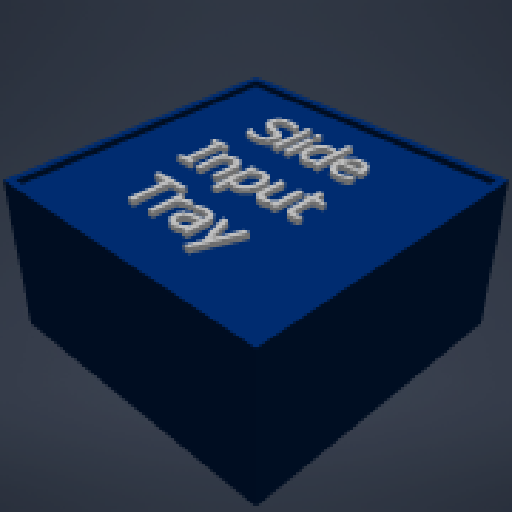
# Autodesk Inventor part: Slide Export Tray
Saved by Autodesk Inventor 2025.1 (Build 291241000, 241)
## iProperties
Created: 2024-10-31
Part Number: Slide Export Tray
Material: Generic
Document SubType Name: Modeling
Designer: jerem
Density: 1 g/cm^3
Appearance: Default
Author: jerem
Autodesk Inventor part; units mm, degrees
ref_plane "YZ Plane" through (0, 0, 0) normal (1, 0, 0) x (0, 1, 0)
ref_plane "XZ Plane" through (0, 0, 0) normal (0, 1, 0) x (-1, 0, 0)
ref_plane "XY Plane" through (0, 0, 0) normal (0, 0, 1) x (1, 0, 0)
sketch "Sketch1" plane through (0, 0, 0) normal (0, 1, 0) x (-1, 0, 0)
  line L0 (-50, 50) -> (50, 50)
  line L1 (50, 50) -> (50, -50)
  line L2 (50, -50) -> (-50, -50)
  line L3 (-50, -50) -> (-50, 50)
  line L4 (-50, 50) -> (50, -50) construction
  line L5 (50, 50) -> (-50, -50) construction
  line L6 (-47.5, 47.5) -> (47.5, 47.5)
  line L7 (47.5, 47.5) -> (47.5, -47.5)
  line L8 (47.5, -47.5) -> (-47.5, -47.5)
  line L9 (-47.5, -47.5) -> (-47.5, 47.5)
  line L10 (-47.5, 47.5) -> (47.5, -47.5) construction
  line L11 (47.5, 47.5) -> (-47.5, -47.5) construction
  point P0 (0, 0)
  dimension "d0" = 100
  dimension "d1" = 100
  dimension "d3" = 95
  constraints: 24 end point, 4 midpoint, 4 parallel, 2 horizontal, 2 perpendicular, 1 point on line
  measures "d0" distance of L1.end L2.end
  measures "d1" distance of L0.end L1.end
  measures "d3" distance of L7.end L8.end
extrude "Extrusion1" add sketch "Sketch1" along normal blind 50 contours L0 L1 L2 L3 | L6 L7 L8 L9
extrude "Extrusion2" add sketch "Sketch1" along normal blind 2 from surface at 50
sketch "Sketch2" plane through (0, 50, 0) normal (0, 1, 0) x (1, 0, 0)
  line L0 (-37.0883, 25.1556) -> (31.9282, 25.1556) construction
  line L1 (31.9282, 25.1556) -> (31.9282, -26.4456) construction
  line L2 (31.9282, -26.4456) -> (-37.0883, -26.4456) construction
  line L3 (-37.0883, -26.4456) -> (-37.0883, 25.1556) construction
  spline S0 degree 2 poles (-18.4674, 18.0229) (-20.0963, 18.0229) (-22.3815, 18.7036) (-23.3904, 19.1899) knots 0 0 0 1 2 2 2
  line L4 (-23.3904, 19.1899) -> (-23.3904, 21.6939)
  line L5 (-23.3904, 21.6939) -> (-23.2446, 21.6939)
  spline S1 degree 2 poles (-23.2446, 21.6939) (-22.26, 20.7701) (-19.7681, 19.749) (-18.6133, 19.749) knots 0 0 0 1 2 2 2
  spline S2 degree 2 poles (-18.6133, 19.749) (-16.9601, 19.749) (-15.2705, 21.1226) (-15.2705, 22.2531) knots 0 0 0 1 2 2 2
  spline S3 degree 2 poles (-15.2705, 22.2531) (-15.2705, 23.1526) (-16.1579, 24.2709) (-17.1181, 24.5505) knots 0 0 0 1 2 2 2
  spline S4 degree 2 poles (-17.1181, 24.5505) (-17.811, 24.745) (-18.9658, 25.0124) (-19.8288, 25.2312) knots 0 0 0 1 2 2 2
  spline S5 degree 2 poles (-19.8288, 25.2312) (-20.6068, 25.4378) (-21.8345, 26.0578) (-22.3086, 26.5561) knots 0 0 0 1 2 2 2
  spline S6 degree 2 poles (-22.3086, 26.5561) (-22.7705, 27.0545) (-23.281, 28.3916) (-23.281, 29.2668) knots 0 0 0 1 2 2 2
  spline S7 degree 2 poles (-23.281, 29.2668) (-23.281, 31.0902) (-20.4366, 33.5578) (-18.2365, 33.5578) knots 0 0 0 1 2 2 2
  spline S8 degree 2 poles (-18.2365, 33.5578) (-16.9723, 33.5578) (-14.7356, 33.0594) (-13.7754, 32.5853) knots 0 0 0 1 2 2 2
  line L6 (-13.7754, 32.5853) -> (-13.7754, 30.2028)
  line L7 (-13.7754, 30.2028) -> (-13.9212, 30.2028)
  spline S9 degree 2 poles (-13.9212, 30.2028) (-14.6384, 30.8592) (-16.875, 31.8317) (-18.1027, 31.8317) knots 0 0 0 1 2 2 2
  spline S10 degree 2 poles (-18.1027, 31.8317) (-19.4885, 31.8317) (-21.2024, 30.531) (-21.2024, 29.4735) knots 0 0 0 1 2 2 2
  spline S11 degree 2 poles (-21.2024, 29.4735) (-21.2024, 28.5253) (-20.1935, 27.3949) (-19.2454, 27.1396) knots 0 0 0 1 2 2 2
  spline S12 degree 2 poles (-19.2454, 27.1396) (-18.6133, 26.9694) (-16.7778, 26.5318) (-16.17, 26.3495) knots 0 0 0 1 2 2 2
  spline S13 degree 2 poles (-16.17, 26.3495) (-14.6262, 25.8754) (-13.1919, 23.967) (-13.1919, 22.5691) knots 0 0 0 1 2 2 2
  spline S14 degree 2 poles (-13.1919, 22.5691) (-13.1919, 21.6818) (-13.9091, 19.98) (-14.5533, 19.3843) knots 0 0 0 1 2 2 2
  spline S15 degree 2 poles (-14.5533, 19.3843) (-15.2705, 18.7279) (-17.0938, 18.0229) (-18.4674, 18.0229) knots 0 0 0 1 2 2 2
  line L8 (-9.375, 18.2903) -> (-11.2713, 18.2903)
  line L9 (-11.2713, 18.2903) -> (-11.2713, 33.9589)
  line L10 (-11.2713, 33.9589) -> (-9.375, 33.9589)
  line L11 (-9.375, 33.9589) -> (-9.375, 18.2903)
  line L12 (-4.6587, 18.2903) -> (-6.5549, 18.2903)
  line L13 (-6.5549, 18.2903) -> (-6.5549, 29.5464)
  line L14 (-6.5549, 29.5464) -> (-4.6587, 29.5464)
  line L15 (-4.6587, 29.5464) -> (-4.6587, 18.2903)
  line L16 (-4.525, 31.4184) -> (-6.6765, 31.4184)
  line L17 (-6.6765, 31.4184) -> (-6.6765, 33.3876)
  line L18 (-6.6765, 33.3876) -> (-4.525, 33.3876)
  line L19 (-4.525, 33.3876) -> (-4.525, 31.4184)
  line L20 (6.7797, 18.2903) -> (4.8835, 18.2903)
  line L21 (4.8835, 18.2903) -> (4.8835, 19.433)
  spline S16 degree 2 poles (4.8835, 19.433) (4.4459, 19.0683) (3.8016, 18.5821) (3.364, 18.3754) knots 0 0 0 1 2 2 2
  spline S17 degree 2 poles (3.364, 18.3754) (2.9629, 18.1809) (2.0998, 17.9743) (1.5285, 17.9743) knots 0 0 0 1 2 2 2
  spline S18 degree 2 poles (1.5285, 17.9743) (0.6047, 17.9743) (-0.9512, 18.7401) (-1.4982, 19.4816) knots 0 0 0 1 2 2 2
  spline S19 degree 2 poles (-1.4982, 19.4816) (-2.0452, 20.2231) (-2.653, 22.4111) (-2.653, 23.8333) knots 0 0 0 1 2 2 2
  spline S20 degree 2 poles (-2.653, 23.8333) (-2.653, 25.3163) (-1.8872, 27.48) (-1.2186, 28.2944) knots 0 0 0 1 2 2 2
  spline S21 degree 2 poles (-1.2186, 28.2944) (-0.5987, 29.0237) (1.1396, 29.8625) (2.0998, 29.8625) knots 0 0 0 1 2 2 2
  spline S22 degree 2 poles (2.0998, 29.8625) (2.9386, 29.8625) (4.1906, 29.4856) (4.8835, 29.0967) knots 0 0 0 1 2 2 2
  line L22 (4.8835, 29.0967) -> (4.8835, 33.9589)
  line L23 (4.8835, 33.9589) -> (6.7797, 33.9589)
  line L24 (6.7797, 33.9589) -> (6.7797, 18.2903)
  line L25 (4.8835, 21.0253) -> (4.8835, 27.5286)
  spline S23 degree 2 poles (4.8835, 27.5286) (4.1785, 27.8689) (3.0601, 28.1242) (2.4159, 28.1242) knots 0 0 0 1 2 2 2
  spline S24 degree 2 poles (2.4159, 28.1242) (0.9572, 28.1242) (-0.6959, 25.9362) (-0.6959, 23.8698) knots 0 0 0 1 2 2 2
  spline S25 degree 2 poles (-0.6959, 23.8698) (-0.6959, 21.8762) (0.5682, 19.7733) (1.9661, 19.7733) knots 0 0 0 1 2 2 2
  spline S26 degree 2 poles (1.9661, 19.7733) (2.7076, 19.7733) (4.2149, 20.454) (4.8835, 21.0253) knots 0 0 0 1 2 2 2
  spline S27 degree 2 poles (14.4135, 18.0351) (11.7149, 18.0351) (8.749, 21.0618) (8.749, 23.8576) knots 0 0 0 1 2 2 2
  spline S28 degree 2 poles (8.749, 23.8576) (8.749, 26.6048) (11.6298, 29.8625) (13.9515, 29.8625) knots 0 0 0 1 2 2 2
  spline S29 degree 2 poles (13.9515, 29.8625) (14.9969, 29.8625) (16.6136, 29.2547) (17.2092, 28.6104) knots 0 0 0 1 2 2 2
  spline S30 degree 2 poles (17.2092, 28.6104) (17.817, 27.9662) (18.4613, 26.1064) (18.4613, 24.7571) knots 0 0 0 1 2 2 2
  line L26 (18.4613, 24.7571) -> (18.4613, 23.7239)
  line L27 (18.4613, 23.7239) -> (10.6695, 23.7239)
  spline S31 degree 2 poles (10.6695, 23.7239) (10.6695, 21.7668) (12.6387, 19.6882) (14.3891, 19.6882) knots 0 0 0 1 2 2 2
  spline S32 degree 2 poles (14.3891, 19.6882) (15.0091, 19.6882) (16.2125, 19.9678) (16.6987, 20.1866) knots 0 0 0 1 2 2 2
  spline S33 degree 2 poles (16.6987, 20.1866) (17.2092, 20.4297) (17.9143, 20.8552) (18.1452, 21.0497) knots 0 0 0 1 2 2 2
  line L28 (18.1452, 21.0497) -> (18.2546, 21.0497)
  line L29 (18.2546, 21.0497) -> (18.2546, 18.9832)
  spline S34 degree 2 poles (18.2546, 18.9832) (17.9264, 18.8495) (16.9297, 18.4605) (16.5407, 18.3511) knots 0 0 0 1 2 2 2
  spline S35 degree 2 poles (16.5407, 18.3511) (15.9937, 18.1931) (15.0942, 18.0351) (14.4135, 18.0351) knots 0 0 0 1 2 2 2
  spline S36 degree 2 poles (16.6136, 25.1704) (16.5893, 25.9362) (16.2733, 27.0545) (15.9694, 27.4313) knots 0 0 0 1 2 2 2
  spline S37 degree 2 poles (15.9694, 27.4313) (15.6412, 27.8568) (14.6079, 28.3065) (13.8421, 28.3065) knots 0 0 0 1 2 2 2
  spline S38 degree 2 poles (13.8421, 28.3065) (13.0885, 28.3065) (12.031, 27.8568) (11.5934, 27.4192) knots 0 0 0 1 2 2 2
  spline S39 degree 2 poles (11.5934, 27.4192) (11.1679, 26.9694) (10.7303, 25.8876) (10.6695, 25.1704) knots 0 0 0 1 2 2 2
  line L30 (10.6695, 25.1704) -> (16.6136, 25.1704)
  line L31 (-20.3333, -6.4068) -> (-26.1437, -6.4068)
  line L32 (-26.1437, -6.4068) -> (-26.1437, -4.8752)
  line L33 (-26.1437, -4.8752) -> (-24.2352, -4.8752)
  line L34 (-24.2352, -4.8752) -> (-24.2352, 7.0616)
  line L35 (-24.2352, 7.0616) -> (-26.1437, 7.0616)
  line L36 (-26.1437, 7.0616) -> (-26.1437, 8.5932)
  line L37 (-26.1437, 8.5932) -> (-20.3333, 8.5932)
  line L38 (-20.3333, 8.5932) -> (-20.3333, 7.0616)
  line L39 (-20.3333, 7.0616) -> (-22.2417, 7.0616)
  line L40 (-22.2417, 7.0616) -> (-22.2417, -4.8752)
  line L41 (-22.2417, -4.8752) -> (-20.3333, -4.8752)
  line L42 (-20.3333, -4.8752) -> (-20.3333, -6.4068)
  line L43 (-9.1745, -6.4068) -> (-11.0707, -6.4068)
  line L44 (-11.0707, -6.4068) -> (-11.0707, 0.0114)
  spline S40 degree 2 poles (-11.0707, 0.0114) (-11.0707, 0.7893) (-11.2166, 2.1265) (-11.4354, 2.5276) knots 0 0 0 1 2 2 2
  spline S41 degree 2 poles (-11.4354, 2.5276) (-11.6664, 2.953) (-12.4929, 3.3663) (-13.198, 3.3663) knots 0 0 0 1 2 2 2
  spline S42 degree 2 poles (-13.198, 3.3663) (-13.903, 3.3663) (-15.3981, 2.6127) (-16.1153, 2.0049) knots 0 0 0 1 2 2 2
  line L45 (-16.1153, 2.0049) -> (-16.1153, -6.4068)
  line L46 (-16.1153, -6.4068) -> (-18.0116, -6.4068)
  line L47 (-18.0116, -6.4068) -> (-18.0116, 4.8493)
  line L48 (-18.0116, 4.8493) -> (-16.1153, 4.8493)
  line L49 (-16.1153, 4.8493) -> (-16.1153, 3.5973)
  spline S43 degree 2 poles (-16.1153, 3.5973) (-15.2644, 4.3631) (-13.6234, 5.1654) (-12.6996, 5.1654) knots 0 0 0 1 2 2 2
  spline S44 degree 2 poles (-12.6996, 5.1654) (-11.0464, 5.1654) (-9.1745, 2.9774) (-9.1745, 0.8987) knots 0 0 0 1 2 2 2
  line L50 (-9.1745, 0.8987) -> (-9.1745, -6.4068)
  spline S45 degree 2 poles (2.9203, -0.4748) (2.9203, -3.2949) (0.234, -6.6256) (-1.8203, -6.6256) knots 0 0 0 1 2 2 2
  spline S46 degree 2 poles (-1.8203, -6.6256) (-2.6591, -6.6256) (-3.9476, -6.2366) (-4.6161, -5.8355) knots 0 0 0 1 2 2 2
  line L51 (-4.6161, -5.8355) -> (-4.6161, -10.5518)
  line L52 (-4.6161, -10.5518) -> (-6.5124, -10.5518)
  line L53 (-6.5124, -10.5518) -> (-6.5124, 4.8493)
  line L54 (-6.5124, 4.8493) -> (-4.6161, 4.8493)
  line L55 (-4.6161, 4.8493) -> (-4.6161, 3.6702)
  spline S47 degree 2 poles (-4.6161, 3.6702) (-3.9111, 4.3145) (-2.185, 5.1654) (-1.1761, 5.1654) knots 0 0 0 1 2 2 2
  spline S48 degree 2 poles (-1.1761, 5.1654) (0.7567, 5.1654) (2.9203, 2.1021) (2.9203, -0.4748) knots 0 0 0 1 2 2 2
  spline S49 degree 2 poles (0.9633, -0.6936) (0.9633, 1.2391) (-0.2644, 3.3663) (-1.638, 3.3663) knots 0 0 0 1 2 2 2
  spline S50 degree 2 poles (-1.638, 3.3663) (-2.4403, 3.3663) (-3.9476, 2.6492) (-4.6161, 2.09) knots 0 0 0 1 2 2 2
  line L56 (-4.6161, 2.09) -> (-4.6161, -4.3038)
  spline S51 degree 2 poles (-4.6161, -4.3038) (-3.8746, -4.6564) (-2.8171, -4.9238) (-2.1364, -4.9238) knots 0 0 0 1 2 2 2
  spline S52 degree 2 poles (-2.1364, -4.9238) (-0.6656, -4.9238) (0.9633, -2.7601) (0.9633, -0.6936) knots 0 0 0 1 2 2 2
  line L57 (13.6416, -6.4068) -> (11.7453, -6.4068)
  line L58 (11.7453, -6.4068) -> (11.7453, -5.1669)
  spline S53 degree 2 poles (11.7453, -5.1669) (10.8701, -5.9327) (9.302, -6.7228) (8.3296, -6.7228) knots 0 0 0 1 2 2 2
  spline S54 degree 2 poles (8.3296, -6.7228) (7.6003, -6.7228) (6.2996, -6.2366) (5.8255, -5.7139) knots 0 0 0 1 2 2 2
  spline S55 degree 2 poles (5.8255, -5.7139) (5.3393, -5.1912) (4.8045, -3.5988) (4.8045, -2.4562) knots 0 0 0 1 2 2 2
  line L59 (4.8045, -2.4562) -> (4.8045, 4.8493)
  line L60 (4.8045, 4.8493) -> (6.7007, 4.8493)
  line L61 (6.7007, 4.8493) -> (6.7007, -1.5688)
  spline S56 degree 2 poles (6.7007, -1.5688) (6.7007, -2.4684) (6.8344, -3.6474) (7.0654, -4.085) knots 0 0 0 1 2 2 2
  spline S57 degree 2 poles (7.0654, -4.085) (7.2964, -4.5226) (8.0865, -4.9238) (8.828, -4.9238) knots 0 0 0 1 2 2 2
  spline S58 degree 2 poles (8.828, -4.9238) (9.5208, -4.9238) (11.0889, -4.1337) (11.7453, -3.5624) knots 0 0 0 1 2 2 2
  line L62 (11.7453, -3.5624) -> (11.7453, 4.8493)
  line L63 (11.7453, 4.8493) -> (13.6416, 4.8493)
  line L64 (13.6416, 4.8493) -> (13.6416, -6.4068)
  spline S59 degree 2 poles (19.7923, -6.6256) (18.2485, -6.6256) (16.5103, -4.863) (16.5103, -2.9546) knots 0 0 0 1 2 2 2
  line L65 (16.5103, -2.9546) -> (16.5103, 3.2812)
  line L66 (16.5103, 3.2812) -> (15.234, 3.2812)
  line L67 (15.234, 3.2812) -> (15.234, 4.8493)
  line L68 (15.234, 4.8493) -> (16.5103, 4.8493)
  line L69 (16.5103, 4.8493) -> (16.5103, 8.0827)
  line L70 (16.5103, 8.0827) -> (18.4066, 8.0827)
  line L71 (18.4066, 8.0827) -> (18.4066, 4.8493)
  line L72 (18.4066, 4.8493) -> (21.8952, 4.8493)
  line L73 (21.8952, 4.8493) -> (21.8952, 3.2812)
  line L74 (21.8952, 3.2812) -> (18.4066, 3.2812)
  line L75 (18.4066, 3.2812) -> (18.4066, -2.0794)
  spline S60 degree 2 poles (18.4066, -2.0794) (18.4066, -2.9303) (18.4673, -3.8662) (18.674, -4.2674) knots 0 0 0 1 2 2 2
  spline S61 degree 2 poles (18.674, -4.2674) (18.8442, -4.6199) (19.61, -4.9724) (20.2664, -4.9724) knots 0 0 0 1 2 2 2
  spline S62 degree 2 poles (20.2664, -4.9724) (20.7283, -4.9724) (21.5913, -4.6928) (21.7858, -4.6077) knots 0 0 0 1 2 2 2
  line L76 (21.7858, -4.6077) -> (21.8952, -4.6077)
  line L77 (21.8952, -4.6077) -> (21.8952, -6.3095)
  spline S63 degree 2 poles (21.8952, -6.3095) (21.3604, -6.4554) (20.2664, -6.6256) (19.7923, -6.6256) knots 0 0 0 1 2 2 2
  line L78 (-17.8536, -31.1039) -> (-17.8536, -17.8786)
  line L79 (-17.8536, -17.8786) -> (-22.886, -17.8786)
  line L80 (-22.886, -17.8786) -> (-22.886, -16.1039)
  line L81 (-22.886, -16.1039) -> (-10.8276, -16.1039)
  line L82 (-10.8276, -16.1039) -> (-10.8276, -17.8786)
  line L83 (-10.8276, -17.8786) -> (-15.86, -17.8786)
  line L84 (-15.86, -17.8786) -> (-15.86, -31.1039)
  line L85 (-15.86, -31.1039) -> (-17.8536, -31.1039)
  line L86 (-3.4856, -21.8778) -> (-3.5829, -21.8778)
  spline S64 degree 2 poles (-3.5829, -21.8778) (-3.8017, -21.817) (-4.2758, -21.7927) (-4.604, -21.7927) knots 0 0 0 1 2 2 2
  spline S65 degree 2 poles (-4.604, -21.7927) (-5.3698, -21.7927) (-6.8771, -22.4612) (-7.5578, -23.1176) knots 0 0 0 1 2 2 2
  line L87 (-7.5578, -23.1176) -> (-7.5578, -31.1039)
  line L88 (-7.5578, -31.1039) -> (-9.454, -31.1039)
  line L89 (-9.454, -31.1039) -> (-9.454, -19.8478)
  line L90 (-9.454, -19.8478) -> (-7.5578, -19.8478)
  line L91 (-7.5578, -19.8478) -> (-7.5578, -21.5253)
  spline S66 degree 2 poles (-7.5578, -21.5253) (-6.5245, -20.6014) (-4.9808, -19.8478) (-4.2515, -19.8478) knots 0 0 0 1 2 2 2
  spline S67 degree 2 poles (-4.2515, -19.8478) (-3.9597, -19.8478) (-3.668, -19.8721) (-3.4856, -19.9086) knots 0 0 0 1 2 2 2
  line L92 (-3.4856, -19.9086) -> (-3.4856, -21.8778)
  spline S68 degree 2 poles (4.2575, -29.9126) (4.0265, -30.0828) (3.2485, -30.6906) (2.8839, -30.8729) knots 0 0 0 1 2 2 2
  spline S69 degree 2 poles (2.8839, -30.8729) (2.3855, -31.1403) (1.4495, -31.4199) (0.5986, -31.4199) knots 0 0 0 1 2 2 2
  spline S70 degree 2 poles (0.5986, -31.4199) (-0.0942, -31.4199) (-1.3463, -30.8972) (-1.8203, -30.4232) knots 0 0 0 1 2 2 2
  spline S71 degree 2 poles (-1.8203, -30.4232) (-2.2701, -29.9612) (-2.8171, -28.5998) (-2.8171, -27.8462) knots 0 0 0 1 2 2 2
  spline S72 degree 2 poles (-2.8171, -27.8462) (-2.8171, -26.6792) (-1.8325, -25.0261) (-0.7628, -24.552) knots 0 0 0 1 2 2 2
  spline S73 degree 2 poles (-0.7628, -24.552) (0.1853, -24.1144) (2.7623, -23.7862) (4.2575, -23.7011) knots 0 0 0 1 2 2 2
  line L93 (4.2575, -23.7011) -> (4.2575, -23.3364)
  spline S74 degree 2 poles (4.2575, -23.3364) (4.2575, -22.68) (3.8563, -21.8656) (3.4917, -21.6347) knots 0 0 0 1 2 2 2
  spline S75 degree 2 poles (3.4917, -21.6347) (3.127, -21.4037) (2.0816, -21.2578) (1.5225, -21.2578) knots 0 0 0 1 2 2 2
  spline S76 degree 2 poles (1.5225, -21.2578) (0.8661, -21.2578) (-0.9087, -21.6468) (-1.796, -22.0236) knots 0 0 0 1 2 2 2
  line L94 (-1.796, -22.0236) -> (-1.9054, -22.0236)
  line L95 (-1.9054, -22.0236) -> (-1.9054, -20.0909)
  spline S77 degree 2 poles (-1.9054, -20.0909) (-1.3827, -19.945) (0.5743, -19.5804) (1.5346, -19.5804) knots 0 0 0 1 2 2 2
  spline S78 degree 2 poles (1.5346, -19.5804) (2.7015, -19.5804) (4.2939, -19.945) (4.926, -20.4191) knots 0 0 0 1 2 2 2
  spline S79 degree 2 poles (4.926, -20.4191) (5.546, -20.881) (6.1537, -22.3518) (6.1537, -23.4094) knots 0 0 0 1 2 2 2
  line L96 (6.1537, -23.4094) -> (6.1537, -31.1039)
  line L97 (6.1537, -31.1039) -> (4.2575, -31.1039)
  line L98 (4.2575, -31.1039) -> (4.2575, -29.9126)
  line L99 (4.2575, -28.3324) -> (4.2575, -25.2084)
  spline S80 degree 2 poles (4.2575, -25.2084) (3.5767, -25.2692) (1.5225, -25.4758) (0.8782, -25.6703) knots 0 0 0 1 2 2 2
  spline S81 degree 2 poles (0.8782, -25.6703) (0.1246, -25.9013) (-0.86, -26.8616) (-0.86, -27.7125) knots 0 0 0 1 2 2 2
  spline S82 degree 2 poles (-0.86, -27.7125) (-0.86, -28.6849) (0.234, -29.6695) (1.2793, -29.6695) knots 0 0 0 1 2 2 2
  spline S83 degree 2 poles (1.2793, -29.6695) (2.1667, -29.6695) (3.6254, -28.9037) (4.2575, -28.3324) knots 0 0 0 1 2 2 2
  line L100 (17.6529, -19.8478) -> (11.5994, -35.2489)
  line L101 (11.5994, -35.2489) -> (9.5695, -35.2489)
  line L102 (9.5695, -35.2489) -> (11.5873, -30.5569)
  line L103 (11.5873, -30.5569) -> (7.503, -19.8478)
  line L104 (7.503, -19.8478) -> (9.5451, -19.8478)
  line L105 (9.5451, -19.8478) -> (12.6205, -28.1865)
  line L106 (12.6205, -28.1865) -> (15.6837, -19.8478)
  line L107 (15.6837, -19.8478) -> (17.6529, -19.8478)
  point P0 (0, 0)
  constraints: 2 other
extrude "Extrusion3" add sketch "Sketch2" along normal blind 2
body "Solid1"
